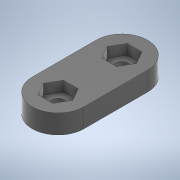
# Autodesk Inventor part: 08-02-01-006_PSBSpacer
Saved by Autodesk Inventor 2020 (Build 240168000, 168)
## iProperties
Created: 2021-07-28
Part Number: 08-02-01-006_PSBSpacer
Material: ABS-Kunststoff(1)
Document SubType Name: Modeling
Designer: Eric
Density: 1.06 g/cm^3
Appearance: Glatt - Weiß(1)
Author: Eric
## iProperties of the stored document _3D-Druck.ipt
Created: 2021-08-26
Part Number: _3D-Druck
Material: Generisch
Document SubType Name: Modeling
Designer: Eric
Density: 1 g/cm^3
Appearance: Vorgabe
Author: Eric
Autodesk Inventor part; units mm, degrees
ref_plane "YZ Plane" through (0, 0, 0) normal (1, 0, 0) x (0, 1, 0)
ref_plane "XZ Plane" through (0, 0, 0) normal (0, 1, 0) x (-1, 0, 0)
ref_plane "XY Plane" through (0, 0, 0) normal (0, 0, 1) x (1, 0, 0)
sketch "Skizze1" plane through (0, 0, 0) normal (0, 1, 0) x (-1, 0, 0)
  circle A0 centre (0, 5) radius 1.05
  circle A1 centre (0, -5) radius 1.05
  line L0 (0, 5) -> (0, -5) construction
  line L1 (0, 5) -> (0, -5) construction
  line L2 (-4.05, 5) -> (-4.05, -5)
  line L3 (4.05, -5) -> (4.05, 5)
  arc A2 (4.05, 5) -> (-4.05, 5) centre (0, 5) ccw
  arc A3 (-4.05, -5) -> (4.05, -5) centre (0, -5) ccw
  point P0 (0, 0)
  point P1 (0, 0)
  point P2 (0, 0)
  dimension "d0" = 2.1
  dimension "d1" = 10
  dimension "d2" = 3
  constraints: 10 end point, 4 centre point, 4 point on circle, 4 tangent, 2 midpoint, 2 vertical, 1 coincident, 1 equal radius, 1 parallel
  measures "d0" diameter of A1
  measures "d1" distance of L0.start L0.end
  measures "d2" radial gap between concentric circles of A3 A1
extrude "Extrusion1" add sketch "Skizze1" along normal blind 3
sketch "Skizze2" plane through (0, 3, 0) normal (0, 1, 0) x (1, 0, 0)
  circle A0 centre (0, 5) radius 1.05 projected
  line L0 (2.3094, 5) -> (1.1547, 3)
  line L1 (1.1547, 3) -> (-1.1547, 3)
  line L2 (-1.1547, 3) -> (-2.3094, 5)
  line L3 (-2.3094, 5) -> (-1.1547, 7)
  line L4 (-1.1547, 7) -> (1.1547, 7)
  line L5 (1.1547, 7) -> (2.3094, 5)
  circle A1 centre (0, -5) radius 1.05 projected
  line L6 (1.1547, -3) -> (2.3094, -5)
  line L7 (2.3094, -5) -> (1.1547, -7)
  line L8 (1.1547, -7) -> (-1.1547, -7)
  line L9 (-1.1547, -7) -> (-2.3094, -5)
  line L10 (-2.3094, -5) -> (-1.1547, -3)
  line L11 (-1.1547, -3) -> (1.1547, -3)
  point P0 (0, 0)
  dimension "d5" = 4
  constraints: 24 end point, 2 coincident, 2 horizontal, 1 parallel, 26 other
  measures "d5" distance between parallel lines of L5 L2
extrude "Extrusion2" cut sketch "Skizze2" against normal blind 1.6
sketch "Skizze3" plane through (0, 0, 0) normal (0, -1, 0) x (1, 0, 0)
  circle A0 centre (0, -5) radius 1.05 projected
  circle A1 centre (0, -5) radius 1.5
  circle A2 centre (0, 5) radius 1.05 projected
  circle A3 centre (0, 5) radius 1.5
  point P0 (0, 0)
  dimension "d8" = 3
  constraints: 2 centre point, 2 coincident, 1 equal radius
  measures "d8" diameter of A1
extrude "Extrusion3" add sketch "Skizze3" along normal blind 1.5
